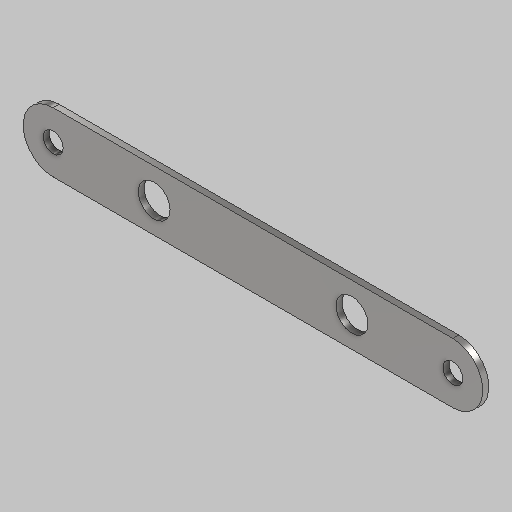
# Autodesk Inventor part: Base - Batentes
Saved by Autodesk Inventor 2025.2 (Build 292293000, 293)
## iProperties
Created: 2024-05-02
Part Number: Base - Batentes
Material: Genérico
Document SubType Name: Modeling
Designer: phmca
Density: 1 g/cm^3
Appearance: Padrão
Author: phmca
Autodesk Inventor part; units mm, degrees
ref_plane "YZ Plane" through (0, 0, 0) normal (1, 0, 0) x (0, 1, 0)
ref_plane "XZ Plane" through (0, 0, 0) normal (0, 1, 0) x (-1, 0, 0)
ref_plane "XY Plane" through (0, 0, 0) normal (0, 0, 1) x (1, 0, 0)
sketch "Esboço1" plane through (0, 0, 0) normal (0, 0, 1) x (1, 0, 0)
  line L0 (-100, 0) -> (100, 0) construction
  line L1 (-100, -15) -> (100, -15)
  line L2 (100, 15) -> (-100, 15)
  arc A0 (-100, 15) -> (-100, -15) centre (-100, 0) ccw
  arc A1 (100, -15) -> (100, 15) centre (100, 0) ccw
  circle A2 centre (-49.5, 0) radius 8
  circle A3 centre (-100, 0) radius 5
  circle A4 centre (49.5, 0) radius 8
  circle A5 centre (100, 0) radius 5
  line L3 (-49.5, 0) -> (49.5, 0)
  line L4 (0, 0) -> (0, 8) construction
  line L5 (0, 0) -> (0, 24.2657) construction
  point P0 (115, 0)
  point P1 (-115, 0)
  dimension "d1" = 16
  dimension "d2" = 10
  dimension "d3" = 16
  dimension "d4" = 10
  dimension "d5" = 99
  dimension "d7" = 30
  dimension "d10" = 200
  constraints: 14 end point, 6 centre point, 6 point on circle, 4 tangent, 2 coincident, 2 collinear, 2 midpoint, 2 point on line, 2 vertical, 1 horizontal, 1 parallel
  measures "d1" diameter of A2
  measures "d2" diameter of A3
  measures "d3" diameter of A4
  measures "d4" diameter of A5
  measures "d5" distance of L3.end L3.start
  measures "d7" distance between parallel lines of L1 L2
  measures "d10" distance of L0.start L0.end
extrude "Extrusão1" add sketch "Esboço1" along normal mid plane 3
sketch "Esboço2" plane through (0, 0, 1.5) normal (0, 0, 1) x (1, 0, 0)
  circle A0 centre (-49.5, 0) radius 8 projected
  line L0 (-41.5, 0) -> (0, 0)
  constraints: 2 end point, 1 horizontal, 1 horizontal alignment, 1 other
sketch "Esboço3" plane through (0, 0, -1.5) normal (0, 0, -1) x (-1, 0, 0)
  circle A0 centre (-49.5, 0) radius 8 projected
  circle A1 centre (49.5, 0) radius 8 projected
  line L0 (-49.5, 0) -> (49.5, 0)
  line L1 (0, 0) -> (0, -45.006)
  constraints: 4 end point, 1 horizontal, 1 vertical
